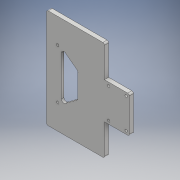
# Autodesk Inventor part: drzaksolaru
Saved by Autodesk Inventor 2017 (Build 210142000, 142)
## iProperties
Created: 2019-02-02
Part Number: drzaksolaru
Material: Generic
Document SubType Name: Modeling
Designer: Denis Kurka
Density: 1 g/cm^3
Appearance: Default
Author: Denis Kurka
Autodesk Inventor part; units mm, degrees
ref_plane "YZ Plane" through (0, 0, 0) normal (1, 0, 0) x (0, 1, 0)
ref_plane "XZ Plane" through (0, 0, 0) normal (0, 1, 0) x (-1, 0, 0)
ref_plane "XY Plane" through (0, 0, 0) normal (0, 0, 1) x (1, 0, 0)
sketch "Sketch1" plane through (0, 0, 0) normal (0, 1, 0) x (-1, 0, 0)
  line L0 (0, 0) -> (70, 0)
  line L1 (70, 0) -> (70, -120)
  line L2 (70, -120) -> (0, -120)
  line L3 (0, -120) -> (0, 0)
  line L4 (0, -82) -> (-30, -82)
  line L5 (-30, -82) -> (-30, -38)
  line L6 (-30, -38) -> (0, -38)
  line L7 (0, -38) -> (0, -82)
  dimension "d0" = 70
  dimension "d1" = 120
  dimension "d2" = 44
  dimension "d3" = 30
  dimension "d4" = 38
  dimension "d5" = 38
  constraints: 16 end point, 4 parallel, 2 horizontal, 2 perpendicular, 1 point on line
  measures "d0" distance of L1.end L2.end
  measures "d1" distance of L0.end L1.end
  measures "d2" distance of L4.end L5.end
  measures "d3" distance of L4.start L4.end
  measures "d4" distance between parallel lines of L0 L6
  measures "d5" distance between parallel lines of L2 L4
extrude "Extrusion1" add sketch "Sketch1" along normal blind 5
sketch "Sketch2" plane through (0, 5, 0) normal (0, 1, 0) x (1, 0, 0)
  line L0 (-67, 3) -> (-3, 3)
  line L1 (-3, 3) -> (-3, 117)
  line L2 (-3, 117) -> (-67, 117)
  line L3 (-67, 117) -> (-67, 3)
  line L4 (-70, 0) -> (0, 0) projected
  line L5 (-70, 120) -> (-70, 0) projected
  line L6 (0, 120) -> (-70, 120) projected
  line L7 (0, 0) -> (0, 38) projected
  dimension "d8" = 3
  dimension "d10" = 3
  dimension "d12" = 3
  dimension "d13" = 3
  constraints: 8 end point, 2 parallel, 1 horizontal, 1 perpendicular
  measures "d8" distance between parallel lines of L4 L0
  measures "d10" distance between parallel lines of L5 L3
  measures "d12" distance between parallel lines of L6 L2
  measures "d13" distance between parallel lines of L7 L1
extrude "Extrusion2" cut sketch "Sketch2" against normal blind 2
sketch "Sketch3" plane through (0, 3, 0) normal (0, 1, 0) x (1, 0, 0)
  line L0 (-52, 30) -> (-52, 90)
  line L1 (-52, 30) -> (-32, 45)
  line L2 (-32, 45) -> (-32, 75)
  line L3 (-32, 75) -> (-52, 90)
  line L4 (-67, 3) -> (-67, 117) projected
  line L5 (-3, 3) -> (-67, 3) projected
  line L6 (-67, 117) -> (-3, 117) projected
  circle A0 centre (-56.4262, 30) radius 1.5
  circle A1 centre (-56.4262, 90) radius 1.5
  point P0 (0, 0)
  dimension "d16" = 60
  dimension "d17" = 30
  dimension "d18" = 15
  dimension "d19" = 20
  dimension "d20" = 42
  dimension "d21" = 42
  dimension "d22" = 27
  dimension "d23" = 27
  dimension "d24" = 3
  dimension "d25" = 3
  dimension "d44" = 27
  dimension "d45" = 27
  constraints: 8 end point, 2 centre point, 1 vertical
  measures "d16" distance of L0.start L0.end
  measures "d17" distance of L1.end L2.end
  measures "d18" distance between parallel lines of L0 L4
  measures "d19" distance between parallel lines of L2 L0
  measures "d20" distance from line of L5 L1.end
  measures "d21" distance from line of L6 L2.end
  measures "d22" distance from line of L5 L0.start
  measures "d23" distance from line of L6 L0.end
  measures "d24" diameter of A0
  measures "d25" diameter of A1
  measures "d44" distance from line of L5 A0.centre
  measures "d45" distance from line of L6 A1.centre
extrude "Extrusion3" cut sketch "Sketch3" against normal blind 10
fillet "Fillet1" radius 3 4 edges at (-52, 1.5, -30) (-32, 1.5, -45) (-32, 1.5, -75) (-52, 1.5, -90)
fillet "Fillet2" radius 2 6 edges at (0, 2.5, 0) (0, 2.5, -120) (-70, 2.5, -120) (-70, 2.5, 0) (30, 2.5, -38) (30, 2.5, -82)
sketch "Sketch4" plane through (0, 5, 0) normal (0, 1, 0) x (1, 0, 0)
  circle A0 centre (26.1, 41.9) radius 1.5
  line L0 (30, 40) -> (30, 80) projected
  line L1 (0, 38) -> (28, 38) projected
  circle A1 centre (26.1, 78.1) radius 1.5
  line L2 (28, 82) -> (0, 82) projected
  circle A2 centre (5.1, 41.9) radius 1.5
  circle A3 centre (5.1, 78.1) radius 1.5
  point P0 (0, 0)
  dimension "d30" = 3
  dimension "d31" = 3.9
  dimension "d32" = 3.9
  dimension "d33" = 3
  dimension "d34" = 3.9
  dimension "d35" = 3.9
  dimension "d36" = 3
  dimension "d37" = 21
  dimension "d38" = 3
  dimension "d39" = 21
  dimension "d40" = 3.9
  dimension "d41" = 3.9
  constraints: 4 centre point
  measures "d30" diameter of A0
  measures "d31" distance from line of L0 A0.centre
  measures "d32" distance from line of A0.centre L1
  measures "d33" diameter of A1
  measures "d34" distance from line of L2 A1.centre
  measures "d35" distance from line of L0 A1.centre
  measures "d36" diameter of A2
  measures "d37" distance of A0.centre A2.centre
  measures "d38" diameter of A3
  measures "d39" distance of A1.centre A3.centre
  measures "d40" distance from line of L2 A3.centre
  measures "d41" distance from line of L1 A2.centre
extrude "Extrusion4" cut sketch "Sketch4" against normal blind 10
equation "\"d4\" = d5"
equation "\"d20\" = d21"
equation "\"d22\" = d23"
equation "\"d44\" = d22"
equation "\"d45\" = d22"
body "Solid1"
